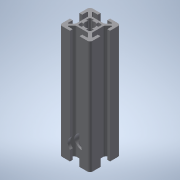
# Autodesk Inventor part: 20x20Profil 1.0
Saved by Autodesk Inventor 2021.3 (Build 253353000, 353)
## iProperties
Created: 2008-10-31
Part Number: 20x20Profil 1.0
Document SubType Name: Modeling
Designer: baerchri
Density: 1 g/cm^3
Material: Allgemein
Appearance: Vorgabe
Author: baerchri
Autodesk Inventor part; units mm, degrees
ref_plane "YZ Plane" through (0, 0, 0) normal (1, 0, 0) x (0, 1, 0)
ref_plane "XZ Plane" through (0, 0, 0) normal (0, 1, 0) x (-1, 0, 0)
ref_plane "XY Plane" through (0, 0, 0) normal (0, 0, 1) x (1, 0, 0)
sketch "Skizze1" plane through (0, 0, 0) normal (0, 0, 1) x (1, 0, 0)
  arc A0 (-6.5142, -3.2) -> (-4.9142, -4.8) centre (-4.9142, -3.2) ccw
  line L0 (-4.9142, -4.8) -> (0.3858, -4.8)
  line L1 (0.3858, -4.8) -> (0.3858, -3)
  line L2 (0.3858, -3) -> (-2.6899, -3)
  arc A1 (-2.9021, -2.4879) -> (-2.6899, -3) centre (-2.69, -2.7) ccw
  line L3 (-2.9021, -2.4879) -> (-0.7071, -0.2929)
  arc A2 (0, 0) -> (-0.7071, -0.2929) centre (0, -1) ccw
  line L4 (0, 0) -> (6.9716, 0)
  arc A3 (7.6787, -0.2929) -> (6.9716, 0) centre (6.9716, -1) ccw
  line L5 (7.6787, -0.2929) -> (9.8737, -2.4879)
  arc A4 (9.6615, -3) -> (9.8737, -2.4879) centre (9.6615, -2.7) ccw
  line L6 (9.6615, -3) -> (6.5858, -3)
  line L7 (6.5858, -3) -> (6.5858, -4.8)
  line L8 (6.5858, -4.8) -> (11.8858, -4.8)
  arc A5 (11.8858, -4.8) -> (13.4858, -3.2) centre (11.8858, -3.2) ccw
  line L9 (13.4858, -3.2) -> (13.4858, 2.1)
  line L10 (13.4858, 2.1) -> (11.6858, 2.1)
  line L11 (11.6858, 2.1) -> (11.6858, -0.9757)
  arc A6 (11.1737, -1.1879) -> (11.6858, -0.9757) centre (11.3858, -0.9757) ccw
  line L12 (11.1737, -1.1879) -> (8.9787, 1.0071)
  arc A7 (8.6858, 1.7142) -> (8.9787, 1.0071) centre (9.6858, 1.7142) ccw
  line L13 (8.6858, 1.7142) -> (8.6858, 8.6858)
  arc A8 (8.9787, 9.3929) -> (8.6858, 8.6858) centre (9.6858, 8.6858) ccw
  line L14 (8.9787, 9.3929) -> (11.1737, 11.5879)
  arc A9 (11.6858, 11.3757) -> (11.1737, 11.5879) centre (11.3858, 11.3757) ccw
  line L15 (11.6858, 11.3757) -> (11.6858, 8.3)
  line L16 (11.6858, 8.3) -> (13.4858, 8.3)
  line L17 (13.4858, 8.3) -> (13.4858, 13.6)
  arc A10 (13.4858, 13.6) -> (11.8858, 15.2) centre (11.8858, 13.6) ccw
  line L18 (11.8858, 15.2) -> (6.5858, 15.2)
  line L19 (6.5858, 15.2) -> (6.5858, 13.4)
  line L20 (6.5858, 13.4) -> (9.6615, 13.4)
  arc A11 (9.8737, 12.8879) -> (9.6615, 13.4) centre (9.6615, 13.1) ccw
  line L21 (9.8737, 12.8879) -> (7.6787, 10.6929)
  arc A12 (6.9716, 10.4) -> (7.6787, 10.6929) centre (6.9716, 11.4) ccw
  line L22 (6.9716, 10.4) -> (0, 10.4)
  arc A13 (-0.7071, 10.6929) -> (0, 10.4) centre (0, 11.4) ccw
  line L23 (-0.7071, 10.6929) -> (-2.9021, 12.8879)
  arc A14 (-2.6899, 13.4) -> (-2.9021, 12.8879) centre (-2.69, 13.1) ccw
  line L24 (-2.6899, 13.4) -> (0.3858, 13.4)
  line L25 (0.3858, 13.4) -> (0.3858, 15.2)
  line L26 (0.3858, 15.2) -> (-4.9142, 15.2)
  arc A15 (-4.9142, 15.2) -> (-6.5142, 13.6) centre (-4.9142, 13.6) ccw
  line L27 (-6.5142, 13.6) -> (-6.5142, 8.3)
  line L28 (-6.5142, 8.3) -> (-4.7142, 8.3)
  line L29 (-4.7142, 8.3) -> (-4.7142, 11.3757)
  arc A16 (-4.2021, 11.5879) -> (-4.7142, 11.3757) centre (-4.4142, 11.3757) ccw
  line L30 (-4.2021, 11.5879) -> (-2.0071, 9.3929)
  arc A17 (-1.7142, 8.6858) -> (-2.0071, 9.3929) centre (-2.7142, 8.6858) ccw
  line L31 (-1.7142, 8.6858) -> (-1.7142, 1.7142)
  arc A18 (-2.0071, 1.0071) -> (-1.7142, 1.7142) centre (-2.7142, 1.7142) ccw
  line L32 (-2.0071, 1.0071) -> (-4.2021, -1.1879)
  arc A19 (-4.7142, -0.9757) -> (-4.2021, -1.1879) centre (-4.4142, -0.9757) ccw
  line L33 (-4.7142, -0.9757) -> (-4.7142, 2.1)
  line L34 (-4.7142, 2.1) -> (-6.5142, 2.1)
  line L35 (-6.5142, 2.1) -> (-6.5142, -3.2)
  line L36 (1.9858, 2.4871) -> (1.9858, 1.2)
  line L37 (1.9858, 1.2) -> (0.1631, 1.2)
  arc A20 (-0.5142, 1.8774) -> (0.1631, 1.2) centre (3.4858, 5.2) ccw
  line L38 (-0.5142, 1.8774) -> (-0.5142, 3.7)
  line L39 (-0.5142, 3.7) -> (0.7729, 3.7)
  arc A21 (0.7729, 6.7) -> (0.7729, 3.7) centre (3.4858, 5.2) ccw
  line L40 (0.7729, 6.7) -> (-0.5142, 6.7)
  line L41 (-0.5142, 6.7) -> (-0.5142, 8.5226)
  arc A22 (0.1631, 9.2) -> (-0.5142, 8.5226) centre (3.4858, 5.2) ccw
  line L42 (0.1631, 9.2) -> (1.9858, 9.2)
  line L43 (1.9858, 9.2) -> (1.9858, 7.9129)
  arc A23 (4.9858, 7.9129) -> (1.9858, 7.9129) centre (3.4858, 5.2) ccw
  line L44 (4.9858, 7.9129) -> (4.9858, 9.2)
  line L45 (4.9858, 9.2) -> (6.8084, 9.2)
  arc A24 (7.4858, 8.5226) -> (6.8084, 9.2) centre (3.4858, 5.2) ccw
  line L46 (7.4858, 8.5226) -> (7.4858, 6.7)
  line L47 (7.4858, 6.7) -> (6.1987, 6.7)
  arc A25 (6.1987, 3.7) -> (6.1987, 6.7) centre (3.4858, 5.2) ccw
  line L48 (6.1987, 3.7) -> (7.4858, 3.7)
  line L49 (7.4858, 3.7) -> (7.4858, 1.8774)
  arc A26 (6.8084, 1.2) -> (7.4858, 1.8774) centre (3.4858, 5.2) ccw
  line L50 (6.8084, 1.2) -> (4.9858, 1.2)
  line L51 (4.9858, 1.2) -> (4.9858, 2.4871)
  arc A27 (1.9858, 2.4871) -> (4.9858, 2.4871) centre (3.4858, 5.2) ccw
  constraints: 104 end point, 56 point on circle, 28 centre point
extrude "Extrusion1" add sketch "Skizze1" against normal blind 74
sketch "Skizze4" plane through (6.5858, -4.8, 0) normal (0, -1, 0) x (1, 0, 0)
  line L0 (-6.5858, 0) -> (0.3858, 0) projected
  line L1 (-13.1, 0) -> (-13.1, -74) projected
  line L2 (-6.5858, -74) -> (0.3858, -74) projected
  point P0 (-3.1, -64)
  dimension "d13" = 10
  dimension "d21" = 10
  measures "d13" distance from line of L1 point (-3.1, -64)
  measures "d21" distance from line of L2 point (-3.1, -64)
hole "Bohrung2" at (3.4858, -4.8, -64) direction (0, 1, 0) diameter 9.2 depth 14.5 tip angle 118
